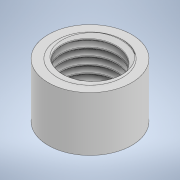
# Autodesk Inventor part: Part4
Saved by Autodesk Inventor 2022.2 (Build 262287000, 287)
## iProperties
Created: 2022-02-06
Part Number: Part4
Material: Generic
Document SubType Name: Modeling
Designer: siwat
Density: 1 g/cm^3
Appearance: Default
Author: siwat
Autodesk Inventor part; units mm, degrees
ref_plane "YZ Plane" through (0, 0, 0) normal (1, 0, 0) x (0, 1, 0)
ref_plane "XZ Plane" through (0, 0, 0) normal (0, 1, 0) x (-1, 0, 0)
ref_plane "XY Plane" through (0, 0, 0) normal (0, 0, 1) x (1, 0, 0)
sketch "Sketch1" plane through (0, 0, 0) normal (0, 1, 0) x (-1, 0, 0)
  circle A0 centre (0, 0) radius 11.5
  circle A1 centre (0, 0) radius 9
  dimension "d0" = 23
  dimension "d1" = 18
  constraints: 2 centre point, 2 coincident
  measures "d0" diameter of A0
  measures "d1" diameter of A1
extrude "Extrusion1" add sketch "Sketch1" along normal blind 15
thread "Thread1" size "M18x2" class "6H" standard "ANSI Metric M Profile" length 15
sketch "Sketch3" plane through (0, 15, 0) normal (1, 0, 0) x (0, 0, 1)
  line L0 (9, 0) -> (9, 15)
  line L1 (9, 15) -> (7.5171, 15)
  line L2 (7.5171, 15) -> (7.5171, 0)
  line L3 (7.5171, 0) -> (9, 0)
  line L4 (0, -5.6171) -> (0, 18.4362) projected
  constraints: 8 end point
revolve "Revolution1" add sketch "Sketch3" angle 360 about axis through (0, 15, 0) along (0, -1, 0) separate body
sketch "Sketch2" plane through (0, 15, 9) normal (-1, 0, 0) x (0, -1, 0)
  line L0 (-1.1668, -0.1013) -> (-1.0001, -0.1013) construction
  line L1 (0.1666, -1.382) -> (-0.0001, -1.7021) construction
  line L2 (-2.0001, -1.7021) -> (-2.1668, -1.382) construction
  line L3 (-0.8334, -0.1013) -> (-1.0001, 0.2189) construction
  line L4 (-1.0001, 0.2189) -> (-1.1668, -0.1013) construction
  line L5 (-2.0001, -1.7021) -> (-1.8334, -1.382) construction
  line L6 (-0.8334, -0.1013) -> (-0.1668, -1.382)
  line L7 (-2.1668, -1.382) -> (-1.8334, -1.382) construction
  arc A0 (-2.1668, -1.382) -> (-2.0001, -1.4831) centre (-2.0001, -1.2952) ccw construction
  line L8 (0.1666, -1.382) -> (-0.1668, -1.382) construction
  line L9 (-2.0001, -1.7021) -> (-2.0001, -1.382) construction
  line L10 (-0.0001, -1.7021) -> (-0.0001, -1.382) construction
  line L11 (-1.0001, 0.2189) -> (-1.0001, -0.0002) construction
  line L12 (-2.0001, -1.4831) -> (-0.0001, -1.4831)
  arc A1 (-2.0001, -1.4831) -> (-1.8334, -1.382) centre (-2.0001, -1.2952) ccw
  line L13 (-0.1668, -1.382) -> (-0.0001, -1.7021) construction
  line L14 (-1.8334, -1.382) -> (-1.1668, -0.1013)
  line L15 (-0.0001, -0.0002) -> (-0.0001, 0.0177)
  line L16 (-0.0001, 0.0177) -> (-0.0001, -0.0002)
  line L17 (-0.0001, -0.0002) -> (0.0334, -0.0002)
  arc A2 (-0.1668, -1.382) -> (-0.0001, -1.4831) centre (-0.0001, -1.2952) ccw
  arc A3 (-0.0001, -1.4831) -> (0.1666, -1.382) centre (-0.0001, -1.2952) ccw construction
  arc A4 (-1.0001, -0.0002) -> (-1.1668, -0.1013) centre (-1.0001, -0.1881) ccw
  arc A5 (-0.8334, -0.1013) -> (-1.0001, -0.0002) centre (-1.0001, -0.1881) ccw
  line L18 (-1.0001, -0.0002) -> (-1.0001, -0.1013) construction
  line L19 (-1.0001, -0.1013) -> (-0.8334, -0.1013) construction
  dimension "d6" = 55
  dimension "d7" = 0.3202
  dimension "d8" = 0.3202
  dimension "Sketch2_ThreadOffset" = 0
  dimension "Sketch2_MajorRadius" = 1.4829
  dimension "d11" = 2
  dimension "Sketch2_MinorRadius" = 0
  constraints: 40 end point, 12 point on circle, 10 parallel, 8 tangent, 6 centre point, 6 collinear, 2 midpoint, 2 point on line, 1 horizontal, 1 perpendicular, 3 other
  measures "d6" angle of L6 L14
  measures "d7" distance of L3.end L0.end
  measures "d8" distance of L1.end L10.end
  measures "Sketch2_ThreadOffset" distance between parallel lines of L15 L10
  measures "Sketch2_MajorRadius" distance from line of L12 L15.start
  measures "d11" distance from line of L1.end L9
  measures "Sketch2_MinorRadius" distance edge to line of A5 L17
coil "Coil1" sketch "Sketch2" operation cut axis through (0, 15, 0) along (0, -1, 0) pitch 2.04 turns 9.313725 hand right bodies 2
equation "\"d6\" = d13"
equation "\"d7\" = 0.160083 * Sketch2_Pitch"
equation "\"d8\" = 0.160083 * Sketch2_Pitch"
equation "\"d11\" = Sketch2_Pitch"
equation "\"d13\" = 55deg"
equation "\"Sketch2_Pitch\" = 2"
body "Solid1"
body "Solid2"
